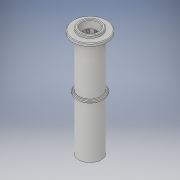
# Autodesk Inventor part: inner_chamber_v9
Saved by Autodesk Inventor 2019 (Build 230136000, 136)
## iProperties
Created: 2021-01-25
Part Number: inner_chamber_v9
Material: Generic
Document SubType Name: Modeling
Designer: wilson
Density: 1 g/cm^3
Appearance: Default
Author: wilson
Autodesk Inventor part; units mm, degrees
ref_plane "YZ Plane" through (0, 0, 0) normal (1, 0, 0) x (0, 1, 0)
ref_plane "XZ Plane" through (0, 0, 0) normal (0, 1, 0) x (-1, 0, 0)
sketch "Sketch1" plane through (0, 0, 0) normal (0, 1, 0) x (-1, 0, 0)
  circle A0 centre (0, 0) radius 4.175
  dimension "d0" = 8.35
  constraints: 1 centre point, 1 coincident
  measures "d0" diameter of A0
extrude "Extrusion1" add sketch "Sketch1" along normal blind 1
sketch "Sketch2" plane through (0, 0, 0) normal (0, -1, 0) x (1, 0, 0)
  circle A0 centre (0, 0) radius 6.5
  dimension "d3" = 13
  constraints: 1 centre point, 1 coincident
  measures "d3" diameter of A0
extrude "Extrusion2" add sketch "Sketch2" along normal blind 1
sketch "Sketch4" plane through (0, -1, 0) normal (0, -1, 0) x (1, 0, 0)
  circle A0 centre (0, 0) radius 4.275
  dimension "d58" = 8.55
  constraints: 1 centre point, 1 coincident
  measures "d58" diameter of A0
extrude "Extrusion3" add sketch "Sketch4" along normal blind 2
ref_plane "Work Plane1" through (0, -1, 0) normal (0, 1, 0) x (1, 0, 0)
sketch "Sketch5" plane through (0, -1, 0) normal (0, 1, 0) x (1, 0, 0)
  point P0 (0, 0)
  point P1 (0, 0)
  constraints: 1 coincident
hole "Hole1" at (0, -1, 0) direction (0, -1, 0) diameter 4.5 depth 391.2125 tip angle 118
sketch "Sketch6" plane through (0, -3, 0) normal (0, -1, 0) x (1, 0, 0)
  line L0 (-0.5, 7.8853) -> (0.5, 7.8853)
  line L1 (0.5, 7.8853) -> (0.5, 1.5409)
  line L2 (0.5, 1.5409) -> (-0.5, 1.5409)
  line L3 (-0.5, 1.5409) -> (-0.5, 7.8853)
  line L4 (-0.5, 7.8853) -> (0.5, 1.5409) construction
  line L5 (0.5, 7.8853) -> (-0.5, 1.5409) construction
  point P0 (0, 0)
  point P1 (0, 4.7131)
  dimension "d17" = 1
  constraints: 12 end point, 2 midpoint, 2 parallel, 1 horizontal, 1 perpendicular
  measures "d17" distance of L1.end L2.end
extrude "Extrusion4" cut sketch "Sketch6" against normal blind 1.5
pattern_circular "Circular Pattern1" count 6 over 360 about axis through (0, -10, 0) along (0, 1, 0) of "Extrusion4"
sketch "Sketch7" plane through (0, -3, 0) normal (0, -1, 0) x (1, 0, 0)
  circle A0 centre (0, 0) radius 4.275
  dimension "d56" = 8.55
  constraints: 1 centre point, 1 coincident
  measures "d56" diameter of A0
extrude "Extrusion5" add sketch "Sketch7" along normal blind 2
sketch "Sketch8" plane through (0, -5, 0) normal (0, -1, 0) x (1, 0, 0)
  circle A0 centre (0, 0) radius 3.175
  line L0 (-3.175, 0) -> (3.175, 0)
  dimension "d25" = 6.35
  constraints: 2 end point, 2 point on circle, 1 centre point, 1 coincident
  measures "d25" diameter of A0
revolve "Revolution2" cut sketch "Sketch8" angle 360 about axis through (-3.175, -5, 0) along (1, 0, 0) picked at (0.7922, 0.7018) contours L0 A0
sketch "Sketch9" plane through (0, 1, 0) normal (0, 1, 0) x (1, 0, 0)
  circle A0 centre (0, 0) radius 3.175
  circle A1 centre (0, 0) radius 3.175 projected
  line L0 (3.175, 0) -> (-3.175, 0)
  constraints: 2 end point, 2 point on circle, 1 centre point, 1 coincident, 1 horizontal
revolve "Revolution3" cut sketch "Sketch9" angle 360 about axis through (3.175, 1, 0) along (-1, 0, 0) picked at (0.7922, 0.7018) contours L0 A0
sketch "Sketch10" plane through (0, -5, 0) normal (0, -1, 0) x (1, 0, 0)
  circle A0 centre (0, 0) radius 4.275
  dimension "d57" = 8.55
  constraints: 1 centre point, 1 coincident
  measures "d57" diameter of A0
extrude "Extrusion6" add sketch "Sketch10" along normal blind 15
sketch "Sketch11" plane through (0, -5, 0) normal (0, 1, 0) x (1, 0, 0)
  point P0 (0, 0)
  point P1 (0, 0)
  constraints: 1 coincident
hole "Hole2" at (0, -5, 0) direction (0, -1, 0) diameter 6.42 depth 391.2125 tip angle 118
sketch "Sketch12" plane through (0, -20, 0) normal (0, -1, 0) x (1, 0, 0)
  circle A0 centre (0, 0) radius 5
  dimension "d37" = 10
  constraints: 1 centre point, 1 coincident
  measures "d37" diameter of A0
extrude "Extrusion7" add sketch "Sketch12" along normal blind 1
sketch "Sketch13" plane through (0, -20, 0) normal (0, 1, 0) x (1, 0, 0)
  point P0 (0, 0)
  point P1 (0, 0)
  constraints: 1 coincident
hole "Hole3" at (0, -20, 0) direction (0, -1, 0) diameter 6.55 depth 391.2125 tip angle 118
sketch "Sketch14" plane through (0, -21, 0) normal (0, -1, 0) x (1, 0, 0)
  circle A0 centre (0, 0) radius 4.275
  dimension "d59" = 8.55
  constraints: 1 centre point, 1 coincident
  measures "d59" diameter of A0
extrude "Extrusion8" add sketch "Sketch14" along normal blind 20
sketch "Sketch15" plane through (0, -21, 0) normal (0, 1, 0) x (1, 0, 0)
  point P0 (0, 0)
  point P1 (0, 0)
  constraints: 1 coincident
hole "Hole4" at (0, -21, 0) direction (0, -1, 0) diameter 6.55 depth 391.2125 tip angle 118
fillet "Fillet1" radius 0.25 3 edges at (0, 1, -3.175) (0, 1, 3.175) (4.175, 1, 0)
sketch "Sketch16" plane through (0, -3, 0) normal (0, 1, 0) x (1, 0, 0)
  circle A0 centre (0, 0) radius 4.275
  dimension "d70" = 8.55
  constraints: 1 centre point, 1 coincident
  measures "d70" diameter of A0
extrude "Extrusion9" add sketch "Sketch16" along normal blind 0.5
sketch "Sketch17" plane through (0, -2.5, 0) normal (0, 1, 0) x (1, 0, 0)
  point P0 (0, 0)
  point P1 (0, 0)
  constraints: 1 coincident
hole "Hole5" at (0, -2.5, 0) direction (0, -1, 0) diameter 4.5 depth 391.2125 tip angle 118
fillet "Fillet2" radius 0.25 2 edges at (-5, -21, 0) (-5, -20, 0)
fillet "Fillet3" radius 0.25 1 edges at (-6.5, 0, 0)
body "Solid1"
